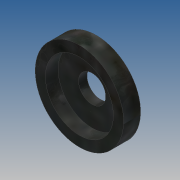
# Autodesk Inventor part: Deckel_ra8846s
Saved by Autodesk Inventor 2021 (Build 250183000, 183)
## iProperties
Created: 2020-12-19
Part Number: Deckel_ra8846s
Material: Stahl
Document SubType Name: Modeling
Designer: Sander
Density: 7.85 g/cm^3
Appearance: Platte
Mass: 0.900309 g
Surface Area: 2.68534 cm^2
Volume: 0.114689 cm^3
Author: Sander
Autodesk Inventor part; units mm, degrees
ref_plane "YZ-Ebene" through (0, 0, 0) normal (1, 0, 0) x (0, 1, 0)
ref_plane "XZ-Ebene" through (0, 0, 0) normal (0, 1, 0) x (-1, 0, 0)
ref_plane "XY-Ebene" through (0, 0, 0) normal (0, 0, 1) x (1, 0, 0)
sketch "Skizze1" plane through (0, 0, 0) normal (0, 0, 1) x (1, 0, 0)
  line L0 (-6.24, 0) -> (1.04, 0) projected
  line L1 (0, -0.5) -> (0, 3) projected
  line L2 (-5.2, 0) -> (-5.2, 2)
  line L3 (-5.2, 2) -> (-3.2, 2.5)
  line L4 (-3.2, 2.5) -> (-1.6, 2.5)
  line L5 (-1.6, 2.5) -> (-1.6, 1.5)
  line L6 (-1.6, 1.5) -> (-4, 1.5)
  line L7 (-4, 1.5) -> (-4, 0)
  point P0 (0, 0)
  dimension "d3" = 3.2
  dimension "d4" = 6.4
  dimension "d5" = 8
  dimension "d6" = 10.4
  dimension "d7" = 2
  dimension "d8" = 2.5
  dimension "d9" = 1.5
  constraints: 12 end point, 4 perpendicular, 2 point on line, 1 vertical
  measures "d3" diameter of L4.end L1
  measures "d4" diameter of L3.end L1
  measures "d5" diameter of L7.end L1
  measures "d6" diameter of L2.start L1
  measures "d7" distance of L2.start L2.end
  measures "d8" distance from line of L0 L3.end
  measures "d9" distance from line of L0 L5.end
revolve "Umdrehung1" add sketch "Skizze1" angle 360 about axis through (0, -10, 0) along (0, 1, 0)
